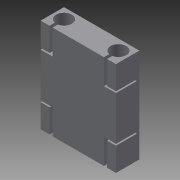
# Autodesk Inventor part: XCarriageHexagon
Saved by Autodesk Inventor 2015 (Build 190159000, 159)
## iProperties
Created: 2014-10-14
Part Number: XCarriageHexagon
Material: Generic
Document SubType Name: Modeling
Designer: Jack
Density: 1 g/cm^3
Appearance: Default
Author: Jack
Autodesk Inventor part; units mm, degrees
ref_plane "YZ Plane" through (0, 0, 0) normal (1, 0, 0) x (0, 1, 0)
ref_plane "XZ Plane" through (0, 0, 0) normal (0, 1, 0) x (-1, 0, 0)
ref_plane "XY Plane" through (0, 0, 0) normal (0, 0, 1) x (1, 0, 0)
sketch "Sketch1" plane through (0, 0, 0) normal (0, 0, 1) x (1, 0, 0)
  line L0 (0, 0) -> (0, 22.35)
  line L1 (0, 22.35) -> (72, 22.35)
  line L2 (72, 22.35) -> (72, 0)
  arc A0 (11.5, 5.0015) -> (8.5, 5.0015) centre (10, 12.35) ccw
  arc A1 (63.5, 5.0015) -> (60.5, 5.0015) centre (62, 12.35) ccw
  line L3 (72, 0) -> (63.5, 0)
  line L4 (63.5, 0) -> (63.5, 5.0015)
  line L5 (60.5, 5.0015) -> (60.5, 0)
  line L6 (60.5, 0) -> (11.5, 0)
  line L7 (11.5, 0) -> (11.5, 5.0015)
  line L8 (8.5, 5.0015) -> (8.5, 0)
  line L9 (8.5, 0) -> (0, 0)
  dimension "d0" = 22.35
  dimension "d1" = 72
  dimension "d2" = 15
  dimension "d4" = 10
  dimension "d5" = 10
  dimension "d6" = 10
  dimension "d7" = 3
  dimension "d8" = 3
  constraints: 20 end point, 5 perpendicular, 4 horizontal alignment, 4 point on circle, 3 point on line, 2 centre point, 2 parallel, 1 equal radius, 1 horizontal, 1 vertical
  measures "d0" distance of L0.start L0.end
  measures "d1" distance of L0.end L1.end
  measures "d2" diameter of A0
  measures "d4" distance from line of L2 A1.centre
  measures "d5" distance from line of L0 A0.centre
  measures "d6" distance from line of L1 A0.centre
  measures "d7" distance between parallel lines of L7 L8
  measures "d8" distance between parallel lines of L4 L5
extrude "Extrusion1" add sketch "Sketch1" along normal blind 90
ref_plane "Work Plane1" through (0, 0, 66) normal (0, 0, 1) x (1, 0, 0)
sketch "Sketch2" plane through (0, 0, 66) normal (0, 0, 1) x (1, 0, 0)
  line L0 (0, 22.35) -> (0, 0) projected
  line L1 (0, 0) -> (8.5, 0) projected
  line L2 (8.5, 0) -> (8.5, 5.0015) projected
  arc A0 (11.5, 5.0015) -> (8.5, 5.0015) centre (10, 12.35) ccw projected
  line L3 (11.5, 5.0015) -> (11.5, 0) projected
  line L4 (11.5, 0) -> (60.5, 0) projected
  line L5 (60.5, 0) -> (60.5, 5.0015) projected
  arc A1 (63.5, 5.0015) -> (60.5, 5.0015) centre (62, 12.35) ccw projected
  line L6 (63.5, 5.0015) -> (63.5, 0) projected
  line L7 (63.5, 0) -> (72, 0) projected
  line L8 (72, 0) -> (72, 22.35) projected
  line L9 (72, 22.35) -> (0, 22.35) projected
  line L10 (8.5, 0) -> (11.5, 0)
  line L11 (11.5, 0) -> (60.5, 0)
  line L12 (60.5, 0) -> (63.5, 0)
  constraints: 6 end point, 2 collinear, 1 horizontal
ref_plane "Work Plane2" through (0, 0, 24) normal (0, 0, -1) x (-1, 0, 0)
extrude "Extrusion2" add sketch "Sketch2" against normal up to surface (42 mm away) contours L2 A0 L3 L10 | L12 L5 A1 L6
sketch "Sketch3" plane through (0, 0, 66) normal (0, 0, 1) x (1, 0, 0)
  arc A0 (11.5, 5.0015) -> (8.5, 5.0015) centre (10, 12.35) ccw projected
  line L0 (60.5, 0) -> (63.5, 0) projected
  line L1 (63.5, 5.0015) -> (63.5, 0) projected
  arc A1 (63.5, 5.0015) -> (60.5, 5.0015) centre (62, 12.35) ccw projected
  line L2 (60.5, 0) -> (60.5, 5.0015) projected
  circle A2 centre (10, 12.35) radius 4.5
  circle A3 centre (62, 12.35) radius 4.5
  point P0 (0, 0)
  dimension "d15" = 9
  dimension "d16" = 9
  constraints: 2 centre point, 2 coincident
  measures "d15" diameter of A2
  measures "d16" diameter of A3
extrude "Extrusion3" cut sketch "Sketch3" against normal up to surface (42 mm away) contours A2 | A3
sketch "Sketch4" plane through (72, 0, 0) normal (1, 0, 0) x (0, 0, -1)
  line L0 (0, 22.35) -> (0, 0) projected
  line L1 (0, 22.35) -> (-90, 22.35) projected
  line L2 (-90, 0) -> (-90, 22.35) projected
  line L3 (0, 0) -> (-90, 0) projected
  line L4 (-66, 5.0015) -> (-66, 19.85) projected
  line L5 (-24, 19.85) -> (-24, 5.0015) projected
  line L6 (-66, 19.85) -> (-67.5, 19.85)
  line L7 (-90, 19.85) -> (-66, 19.85) projected
  line L8 (-67.5, 19.85) -> (-67.5, 0)
  line L9 (0, 0) -> (-90, 0) projected
  line L10 (-66, 5.0015) -> (-66, 0)
  line L11 (-66, 0) -> (-66, 5.0015) projected
  line L12 (-24, 19.85) -> (-22.5, 19.85)
  line L13 (-24, 19.85) -> (0, 19.85) projected
  line L14 (-22.5, 19.85) -> (-22.5, 0)
  line L15 (-24, 5.0015) -> (-24, 0)
  line L16 (-24, 5.0015) -> (-24, 0) projected
  dimension "d19" = 1.5
  dimension "d20" = 1.5
  constraints: 12 end point, 4 point on line, 2 collinear, 2 perpendicular
  measures "d19" distance of L4.end L6.end
  measures "d20" distance of L5.start L12.end
extrude "Extrusion4" cut sketch "Sketch4" against normal blind 10 contours L14 L3 L15 L5 L12 | L6 L4 L10 L3 L8
sketch "Sketch5" plane through (0, 0, 0) normal (-1, 0, 0) x (0, 0, 1)
  line L0 (0, 0) -> (90, 0) projected
  line L1 (67.5, 0) -> (67.5, 19.85) projected
  line L2 (67.5, 19.85) -> (66, 19.85) projected
  line L3 (66, 19.85) -> (66, 0) projected
  line L4 (24, 0) -> (24, 19.85) projected
  line L5 (24, 19.85) -> (22.5, 19.85) projected
  line L6 (22.5, 19.85) -> (22.5, 0) projected
extrude "Extrusion5" cut sketch "Sketch5" against normal blind 10
sketch "Sketch10" plane through (0, 22.35, 0) normal (0, 1, 0) x (1, 0, 0)
  line L0 (0, 0) -> (72, 0) projected
  line L1 (0, 0) -> (0, -90) projected
  line L2 (72, -90) -> (0, -90) projected
  line L3 (26.185, -76) -> (31.0925, -67.5)
  line L4 (31.0925, -67.5) -> (40.9075, -67.5)
  line L5 (40.9075, -67.5) -> (45.815, -76)
  line L6 (45.815, -76) -> (40.9075, -84.5)
  line L7 (40.9075, -84.5) -> (31.0925, -84.5)
  line L8 (31.0925, -84.5) -> (26.185, -76)
  line L9 (26.185, -14) -> (31.0925, -5.5)
  line L10 (31.0925, -5.5) -> (40.9075, -5.5)
  line L11 (40.9075, -5.5) -> (45.815, -14)
  line L12 (45.815, -14) -> (40.9075, -22.5)
  line L13 (40.9075, -22.5) -> (31.0925, -22.5)
  line L14 (31.0925, -22.5) -> (26.185, -14)
  point P0 (36, -76)
  point P1 (36, -14)
  dimension "d43" = 17
  dimension "d44" = 36
  dimension "d45" = 14
  dimension "d46" = 14
  constraints: 24 end point, 2 horizontal, 2 vertical alignment, 26 other
  measures "d43" distance between parallel lines of L4 L7
  measures "d44" distance from line of L1 point (36, -14)
  measures "d45" distance from line of L0 point (36, -14)
  measures "d46" distance from line of L2 point (36, -76)
extrude "Extrusion9" cut sketch "Sketch10" against normal blind 18.35
sketch "Sketch11" plane through (0, 22.35, 0) normal (0, 1, 0) x (1, 0, 0)
  line L0 (26.185, -76) -> (31.0925, -67.5) projected
  line L1 (31.0925, -67.5) -> (40.9075, -67.5) projected
  line L2 (40.9075, -67.5) -> (45.815, -76) projected
  line L3 (31.0925, -22.5) -> (26.185, -14) projected
  line L4 (45.815, -14) -> (40.9075, -22.5) projected
  line L5 (40.9075, -22.5) -> (31.0925, -22.5) projected
  line L6 (0, 0) -> (0, -90) projected
  line L7 (49, -14) -> (49, -76)
  line L8 (49, -76) -> (45.815, -76)
  line L9 (49, -14) -> (45.815, -14)
  line L10 (26.185, -14) -> (23, -14)
  line L11 (23, -14) -> (23, -76)
  line L12 (23, -76) -> (26.185, -76)
  dimension "d49" = 26
  dimension "d50" = 23
  constraints: 12 end point, 3 perpendicular, 2 point on line, 1 parallel, 1 vertical
  measures "d49" distance between parallel lines of L7 L11
  measures "d50" distance between parallel lines of L6 L11
extrude "Extrusion10" cut sketch "Sketch11" against normal up to surface (18.35 mm away)
sketch "Sketch12" plane through (0, 22.35, 0) normal (0, 1, 0) x (1, 0, 0)
  line L0 (0, 0) -> (0, -90) projected
  line L1 (72, -90) -> (0, -90) projected
  circle A0 centre (51, -45) radius 13
  circle A1 centre (21, -45) radius 13
  dimension "d53" = 26
  dimension "d54" = 26
  dimension "d55" = 30
  dimension "d56" = 21
  dimension "d57" = 45
  constraints: 2 centre point, 1 horizontal alignment
  measures "d53" diameter of A0
  measures "d54" diameter of A1
  measures "d55" distance of A0.centre A1.centre
  measures "d56" distance from line of L0 A1.centre
  measures "d57" distance from line of L1 A1.centre
extrude "Extrusion11" cut sketch "Sketch12" against normal blind 2
body "Solid1"
